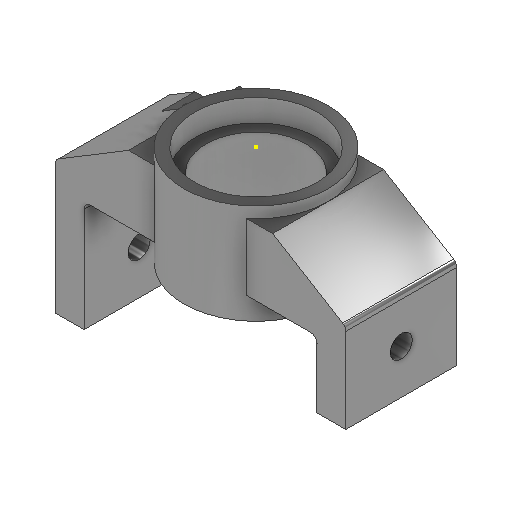
# Autodesk Inventor part: upright2025
Saved by Autodesk Inventor 2025.2 (Build 292293000, 293)
## iProperties
Created: 2025-05-12
Part Number: upright2025
Material: Generic
Document SubType Name: Modeling
Designer: spars
Density: 1 g/cm^3
Appearance: Chrome - Polished Black
Author: spars
Autodesk Inventor part; units mm, degrees
ref_plane "YZ Plane" through (0, 0, 0) normal (1, 0, 0) x (0, 1, 0)
ref_plane "XZ Plane" through (0, 0, 0) normal (0, 1, 0) x (-1, 0, 0)
sketch "Sketch1" plane through (0, 0, 0) normal (0, 0, 1) x (1, 0, 0)
  line L0 (-32.5, 15) -> (32.5, 15)
  line L1 (32.5, 15) -> (32.5, -15)
  line L2 (-32.5, -15) -> (-32.5, 15)
  line L3 (-32.5, 15) -> (32.5, -15) construction
  line L4 (32.5, 15) -> (-32.5, -15) construction
  line L5 (-22.5, 15) -> (11.5921, 15) construction
  line L6 (-22.5, -15) -> (-49.5, -15)
  line L7 (-52.5, -18) -> (-52.5, -65)
  line L8 (-52.5, -65) -> (-65.5, -65)
  line L9 (-65.5, -65) -> (-65.5, -6.6898)
  line L10 (-64.0549, -4.1242) -> (-32.5, 15)
  arc A0 (-64.0549, -4.1242) -> (-65.5, -6.6898) centre (-62.5, -6.6898) ccw
  arc A1 (-49.5, -15) -> (-52.5, -18) centre (-49.5, -18) ccw
  line L11 (32.5, -15) -> (22.5, -15)
  line L12 (32.5, -15) -> (49.5, -15)
  line L13 (52.5, -18) -> (52.5, -45)
  line L14 (52.5, -45) -> (65.5, -45)
  line L15 (65.5, -45) -> (65.5, -6.6898)
  line L16 (64.0549, -4.1242) -> (32.5, 15)
  arc A2 (65.5, -6.6898) -> (64.0549, -4.1242) centre (62.5, -6.6898) ccw
  arc A3 (52.5, -18) -> (49.5, -15) centre (49.5, -18) ccw
  line L17 (-22.5, -15) -> (22.5, -15)
  point P0 (0, 0)
  point P1 (-22.5, -2.0461)
  point P2 (-52.5, -15)
  point P3 (-65.5, -5)
  point P4 (52.5, -15)
  point P5 (65.5, -5)
  dimension "d0" = 65
  dimension "d1" = 30
  dimension "d3" = 10
  dimension "d4" = 30
  dimension "d5" = 50
  dimension "d6" = 13
  dimension "d7" = 60
  dimension "d8" = 3
  dimension "d10" = 20
  dimension "d11" = 30
  dimension "d12" = 13
  dimension "d13" = 40
  dimension "d14" = 3
  constraints: 36 end point, 10 point on line, 8 point on circle, 8 tangent, 7 perpendicular, 4 centre point, 4 horizontal, 2 equal radius, 2 midpoint, 1 parallel
  measures "d0" distance of L1.end L2.start
  measures "d1" distance of L0.end L1.end
  measures "d3" distance from line of L2 point (-22.5, -2.046)
  measures "d4" distance of L6.start point (-52.5, -15)
  measures "d5" distance of point (-52.5, -15) L7.end
  measures "d6" distance of L7.end L8.end
  measures "d7" distance of L8.end point (-65.5, -5)
  measures "d8" radius of A0
  measures "d10" distance of L1.end point (52.5, -15)
  measures "d11" distance of point (52.5, -15) L13.end
  measures "d12" distance of L13.end L14.end
  measures "d13" distance of L14.end point (65.5, -5)
  measures "d14" radius of A2
extrude "Extrusion1" add sketch "Sketch1" along normal mid plane 50
sketch "Sketch2" plane through (-32.5, 15, 25) normal (0, 1, 0) x (1, 0, 0)
  circle A0 centre (32.5, 25) radius 32.5
  dimension "d17" = 65
  constraints: 1 centre point, 1 coincident
  measures "d17" diameter of A0
extrude "Extrusion2" add sketch "Sketch2" along normal blind 5 and the other way blind 40
sketch "Sketch3" plane through (0, 20, 0) normal (0, 1, 0) x (1, 0, 0)
  circle A0 centre (0, 0) radius 27.5
  dimension "d22" = 55
  constraints: 1 centre point, 1 coincident
  measures "d22" diameter of A0
sketch "Sketch4" plane through (0, 20, 0) normal (0, 1, 0) x (1, 0, 0)
  point P0 (0, 0)
extrude "Extrusion3" cut sketch "Sketch3" against normal through all
ref_plane "Work Plane1" through (0, 10, 0) normal (0, 1, 0) x (1, 0, 0)
sketch "Sketch5" plane through (0, 10, 0) normal (0, 1, 0) x (1, 0, 0)
  circle A0 centre (0, 0) radius 27.5
  circle A1 centre (0, 0) radius 22.5
  dimension "d26" = 55
  dimension "d27" = 45
  constraints: 2 centre point, 2 coincident
  measures "d26" diameter of A0
  measures "d27" diameter of A1
extrude "Extrusion4" add sketch "Sketch5" against normal blind 25
sketch "Sketch6" plane through (-65.5, -65, 25) normal (-1, 0, 0) x (0, 0, 1)
  circle A0 centre (-24.7708, 20) radius 5
  line L0 (-50, 0) -> (-50, 58.3102) projected
  line L1 (2.5, 40) -> (-52.5, 40) projected
  line L2 (-50, 0) -> (0.2292, 0)
  line L3 (0.2292, 0) -> (0.2292, 40)
  line L4 (0.2292, 40) -> (-50, 40)
  line L5 (-50, 40) -> (-50, 0)
  point P0 (-25, 65)
  dimension "d30" = 10
  dimension "d31" = 20
  dimension "d33" = 25
  constraints: 8 end point, 2 parallel, 1 centre point, 1 horizontal, 1 perpendicular, 1 point on line, 1 vertical
  measures "d30" diameter of A0
  measures "d31" distance from line of L2 A0.centre
  measures "d33" distance from line of L3 A0.centre
extrude "Extrusion5" cut sketch "Sketch6" against normal blind 25 contours A0
sketch "Sketch7" plane through (65.5, -45, 25) normal (1, 0, 0) x (0, 0, -1)
  circle A0 centre (25, 20) radius 5
  line L0 (50, 0) -> (0, 0) projected
  line L1 (50, 38.3102) -> (50, 0) projected
  point P0 (25, 45)
  dimension "d36" = 10
  dimension "d37" = 20
  dimension "d38" = 25
  constraints: 1 centre point
  measures "d36" diameter of A0
  measures "d37" distance from line of L0 A0.centre
  measures "d38" distance from line of L1 A0.centre
extrude "Extrusion6" cut sketch "Sketch7" against normal blind 20
sketch "Sketch8" plane through (0, 0, -25) normal (0, 0, -1) x (-1, 0, 0)
  line L0 (32.5, 15) -> (64.0549, -4.1242) projected
  line L1 (32.5, 15) -> (32.5, 3)
  line L2 (32.5, 3) -> (52.4996, 2.879)
  point P0 (0, 0)
  dimension "d41" = 12
  dimension "d42" = 20
  constraints: 4 end point, 1 point on line, 1 vertical
  measures "d41" distance of L0.start L1.end
  measures "d42" distance of L1.end L2.end
extrude "Extrusion7" cut sketch "Sketch8" against normal blind 15
sketch "Sketch9" plane through (-52.4996, 2.879, -10) normal (-0.006, 1, 0) x (1, 0.006, 0)
  circle A0 centre (5, 7.5) radius 2.5
  circle A1 centre (15, 7.5) radius 2.5
  line L0 (0, 0) -> (0, 15) projected
  line L1 (20.0726, 15) -> (20.0726, 0) projected
  line L2 (0, 15) -> (20, 15) projected
  point P0 (52.4813, -10)
  dimension "d45" = 5
  dimension "d46" = 5
  dimension "d48" = 10
  dimension "d49" = 5
  dimension "d51" = 7.5
  dimension "d52" = 7.5
  constraints: 2 centre point
  measures "d45" diameter of A0
  measures "d46" diameter of A1
  measures "d48" distance of A0.centre A1.centre
  measures "d49" distance from line of L0 A0.centre
  measures "d51" distance from line of L2 A0.centre
  measures "d52" distance from line of L2 A1.centre
extrude "Extrusion8" cut sketch "Sketch9" against normal blind 25
sketch "Sketch10" plane through (-49.5, -15, -25) normal (0, -1, 0) x (1, 0, 0)
  line L0 (17, 0) -> (17, 15) projected
  line L1 (-2.9996, 15) -> (17, 15) projected
  line L2 (17, 0) -> (-1, 0)
  line L3 (-1, 0) -> (-1, 15)
  line L4 (-1, 15) -> (17, 15)
  line L5 (17, 15) -> (17, 0)
  point P0 (49.5, 25)
  dimension "d55" = 18
  constraints: 8 end point, 2 parallel, 1 horizontal, 1 perpendicular, 1 point on line
  measures "d55" distance of L3.end L4.end
extrude "Extrusion9" cut sketch "Sketch10" against normal blind 5
equation "\"d52\" = d51"
body "Solid1"
